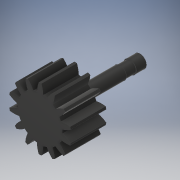
# Autodesk Inventor part: AC06
Saved by Autodesk Inventor 2017 (Build 210142000, 142)
## iProperties
Created: 2019-09-22
Part Number: AC06
Material: ABS Plastic
Document SubType Name: Modeling
Designer: Zach
Density: 1.06 g/cm^3
Appearance: Smooth - Black
Author: Zach
Autodesk Inventor part; units mm, degrees
ref_plane "YZ Plane" through (0, 0, 0) normal (1, 0, 0) x (0, 1, 0)
ref_plane "XZ Plane" through (0, 0, 0) normal (0, 1, 0) x (-1, 0, 0)
ref_plane "XY Plane" through (0, 0, 0) normal (0, 0, 1) x (1, 0, 0)
sketch "Sketch1" plane through (0, 0, 0) normal (0, 0, 1) x (1, 0, 0)
  arc A0 (5.9892, 8.4411) -> (6.9584, 12.5904) centre (-5.202, 13.243) ccw
  arc A1 (6.9584, 12.5904) -> (5.505, 13.2903) centre (0, 0) ccw
  arc A2 (5.505, 13.2903) -> (2.8652, 9.9455) centre (13.5971, 4.1898) ccw
  arc A3 (2.8652, 9.9455) -> (1.7337, 10.2038) centre (0, 0) ccw
  arc A4 (1.7337, 10.2038) -> (0.8066, 14.3627) centre (-10.4327, 9.6744) ccw
  arc A5 (0.8066, 14.3627) -> (-0.8066, 14.3627) centre (0, 0) ccw
  arc A6 (-0.8066, 14.3627) -> (-1.7337, 10.2038) centre (10.4327, 9.6744) ccw
  arc A7 (-1.7337, 10.2038) -> (-2.8652, 9.9455) centre (0, 0) ccw
  arc A8 (-2.8652, 9.9455) -> (-5.505, 13.2903) centre (-13.5971, 4.1898) ccw
  arc A9 (-5.505, 13.2903) -> (-6.9584, 12.5904) centre (0, 0) ccw
  arc A10 (-6.9584, 12.5904) -> (-5.9892, 8.4411) centre (5.202, 13.243) ccw
  arc A11 (-5.9892, 8.4411) -> (-6.8967, 7.7174) centre (0, 0) ccw
  arc A12 (-6.8967, 7.7174) -> (-10.7263, 9.5856) centre (-14.0685, -2.1247) ccw
  arc A13 (-10.7263, 9.5856) -> (-11.7321, 8.3244) centre (0, 0) ccw
  arc A14 (-11.7321, 8.3244) -> (-9.0586, 5.0065) centre (-1.0591, 14.1885) ccw
  arc A15 (-9.0586, 5.0065) -> (-9.5622, 3.9608) centre (0, 0) ccw
  arc A16 (-9.5622, 3.9608) -> (-13.8231, 3.9824) centre (-11.7534, -8.0184) ccw
  arc A17 (-13.8231, 3.9824) -> (-14.1821, 2.4096) centre (0, 0) ccw
  arc A18 (-14.1821, 2.4096) -> (-10.3337, 0.5803) centre (-7.1104, 12.3239) ccw
  arc A19 (-10.3337, 0.5803) -> (-10.3337, -0.5803) centre (0, 0) ccw
  arc A20 (-10.3337, -0.5803) -> (-14.1821, -2.4096) centre (-7.1104, -12.3239) ccw
  arc A21 (-14.1821, -2.4096) -> (-13.8231, -3.9824) centre (0, 0) ccw
  arc A22 (-13.8231, -3.9824) -> (-9.5622, -3.9608) centre (-11.7534, 8.0184) ccw
  arc A23 (-9.5622, -3.9608) -> (-9.0586, -5.0065) centre (0, 0) ccw
  arc A24 (-9.0586, -5.0065) -> (-11.7321, -8.3244) centre (-1.0591, -14.1885) ccw
  arc A25 (-11.7321, -8.3244) -> (-10.7263, -9.5856) centre (0, 0) ccw
  arc A26 (-10.7263, -9.5856) -> (-6.8967, -7.7174) centre (-14.0685, 2.1247) ccw
  arc A27 (-6.8967, -7.7174) -> (-5.9892, -8.4411) centre (0, 0) ccw
  arc A28 (-5.9892, -8.4411) -> (-6.9584, -12.5904) centre (5.202, -13.243) ccw
  arc A29 (-6.9584, -12.5904) -> (-5.505, -13.2903) centre (0, 0) ccw
  arc A30 (-5.505, -13.2903) -> (-2.8652, -9.9455) centre (-13.5971, -4.1898) ccw
  arc A31 (-2.8652, -9.9455) -> (-1.7337, -10.2038) centre (0, 0) ccw
  arc A32 (-1.7337, -10.2038) -> (-0.8066, -14.3627) centre (10.4327, -9.6744) ccw
  arc A33 (-0.8066, -14.3627) -> (0.8066, -14.3627) centre (0, 0) ccw
  arc A34 (0.8066, -14.3627) -> (1.7337, -10.2038) centre (-10.4327, -9.6744) ccw
  arc A35 (1.7337, -10.2038) -> (2.8652, -9.9455) centre (0, 0) ccw
  arc A36 (2.8652, -9.9455) -> (5.505, -13.2903) centre (13.5971, -4.1898) ccw
  arc A37 (5.505, -13.2903) -> (6.9584, -12.5904) centre (0, 0) ccw
  arc A38 (6.9584, -12.5904) -> (5.9892, -8.4411) centre (-5.202, -13.243) ccw
  arc A39 (5.9892, -8.4411) -> (6.8967, -7.7174) centre (0, 0) ccw
  arc A40 (6.8967, -7.7174) -> (10.7263, -9.5856) centre (14.0685, 2.1247) ccw
  arc A41 (10.7263, -9.5856) -> (11.7321, -8.3244) centre (0, 0) ccw
  arc A42 (11.7321, -8.3244) -> (9.0586, -5.0065) centre (1.0591, -14.1885) ccw
  arc A43 (9.0586, -5.0065) -> (9.5622, -3.9608) centre (0, 0) ccw
  arc A44 (9.5622, -3.9608) -> (13.8231, -3.9824) centre (11.7534, 8.0184) ccw
  arc A45 (13.8231, -3.9824) -> (14.1821, -2.4096) centre (0, 0) ccw
  arc A46 (14.1821, -2.4096) -> (10.3337, -0.5803) centre (7.1104, -12.3239) ccw
  arc A47 (10.3337, -0.5803) -> (10.3337, 0.5803) centre (0, 0) ccw
  arc A48 (10.3337, 0.5803) -> (14.1821, 2.4096) centre (7.1104, 12.3239) ccw
  arc A49 (14.1821, 2.4096) -> (13.8231, 3.9824) centre (0, 0) ccw
  arc A50 (13.8231, 3.9824) -> (9.5622, 3.9608) centre (11.7534, -8.0184) ccw
  arc A51 (9.5622, 3.9608) -> (9.0586, 5.0065) centre (0, 0) ccw
  arc A52 (9.0586, 5.0065) -> (11.7321, 8.3244) centre (1.0591, 14.1885) ccw
  arc A53 (11.7321, 8.3244) -> (10.7263, 9.5856) centre (0, 0) ccw
  arc A54 (10.7263, 9.5856) -> (6.8967, 7.7174) centre (14.0685, -2.1247) ccw
  arc A55 (6.8967, 7.7174) -> (5.9892, 8.4411) centre (0, 0) ccw
  constraints: 112 point on circle, 56 centre point
extrude "Extrusion1" add sketch "Sketch1" along normal blind 16
sketch "Sketch2" plane through (0, 0, 0) normal (0, 0, -1) x (-1, 0, 0)
  circle A0 centre (0, 0) radius 2.925
  dimension "d2" = 5.85
  constraints: 1 centre point, 1 coincident
  measures "d2" diameter of A0
extrude "Extrusion2" add sketch "Sketch2" along normal blind 20
sketch "Sketch4" plane through (0, 0, -20) normal (0, 0, -1) x (-1, 0, 0)
  circle A0 centre (0, 0) radius 2.675
  dimension "d8" = 5.35
  constraints: 1 centre point, 1 coincident
  measures "d8" diameter of A0
extrude "Extrusion4" add sketch "Sketch4" along normal blind 4.5
sketch "Sketch7" plane through (0, 0, -24.5) normal (0, 0, -1) x (-1, 0, 0)
  circle A0 centre (0, 0) radius 2.925 projected
extrude "Extrusion6" add sketch "Sketch7" along normal blind 4.5
sketch "Sketch10" plane through (0, 0, 16) normal (0, 0, 1) x (1, 0, 0)
  arc A0 (10.7263, 9.5856) -> (6.8967, 7.7174) centre (14.0685, -2.1247) ccw projected
  arc A1 (6.8967, 7.7174) -> (5.9892, 8.4411) centre (0, 0) ccw projected
  arc A2 (5.9892, 8.4411) -> (6.9584, 12.5904) centre (-5.202, 13.243) ccw projected
  arc A3 (6.9584, 12.5904) -> (5.505, 13.2903) centre (0, 0) ccw projected
  arc A4 (5.505, 13.2903) -> (2.8652, 9.9455) centre (13.5971, 4.1898) ccw projected
  arc A5 (2.8652, 9.9455) -> (1.7337, 10.2038) centre (0, 0) ccw projected
  arc A6 (1.7337, 10.2038) -> (0.8066, 14.3627) centre (-10.4327, 9.6744) ccw projected
  arc A7 (0.8066, 14.3627) -> (-0.8066, 14.3627) centre (0, 0) ccw projected
  arc A8 (-0.8066, 14.3627) -> (-1.7337, 10.2038) centre (10.4327, 9.6744) ccw projected
  arc A9 (-1.7337, 10.2038) -> (-2.8652, 9.9455) centre (0, 0) ccw projected
  arc A10 (-2.8652, 9.9455) -> (-5.505, 13.2903) centre (-13.5971, 4.1898) ccw projected
  arc A11 (-5.505, 13.2903) -> (-6.9584, 12.5904) centre (0, 0) ccw projected
  arc A12 (-6.9584, 12.5904) -> (-5.9892, 8.4411) centre (5.202, 13.243) ccw projected
  arc A13 (-5.9892, 8.4411) -> (-6.8967, 7.7174) centre (0, 0) ccw projected
  arc A14 (-6.8967, 7.7174) -> (-10.7263, 9.5856) centre (-14.0685, -2.1247) ccw projected
  arc A15 (-10.7263, 9.5856) -> (-11.7321, 8.3244) centre (0, 0) ccw projected
  arc A16 (-11.7321, 8.3244) -> (-9.0586, 5.0065) centre (-1.0591, 14.1885) ccw projected
  arc A17 (-9.0586, 5.0065) -> (-9.5622, 3.9608) centre (0, 0) ccw projected
  arc A18 (-9.5622, 3.9608) -> (-13.8231, 3.9824) centre (-11.7534, -8.0184) ccw projected
  arc A19 (-13.8231, 3.9824) -> (-14.1821, 2.4096) centre (0, 0) ccw projected
  arc A20 (-14.1821, 2.4096) -> (-10.3337, 0.5803) centre (-7.1104, 12.3239) ccw projected
  arc A21 (-10.3337, 0.5803) -> (-10.3337, -0.5803) centre (0, 0) ccw projected
  arc A22 (-10.3337, -0.5803) -> (-14.1821, -2.4096) centre (-7.1104, -12.3239) ccw projected
  arc A23 (-14.1821, -2.4096) -> (-13.8231, -3.9824) centre (0, 0) ccw projected
  arc A24 (-13.8231, -3.9824) -> (-9.5622, -3.9608) centre (-11.7534, 8.0184) ccw projected
  arc A25 (-9.5622, -3.9608) -> (-9.0586, -5.0065) centre (0, 0) ccw projected
  arc A26 (-9.0586, -5.0065) -> (-11.7321, -8.3244) centre (-1.0591, -14.1885) ccw projected
  arc A27 (-11.7321, -8.3244) -> (-10.7263, -9.5856) centre (0, 0) ccw projected
  arc A28 (-10.7263, -9.5856) -> (-6.8967, -7.7174) centre (-14.0685, 2.1247) ccw projected
  arc A29 (-6.8967, -7.7174) -> (-5.9892, -8.4411) centre (0, 0) ccw projected
  arc A30 (-5.9892, -8.4411) -> (-6.9584, -12.5904) centre (5.202, -13.243) ccw projected
  arc A31 (-6.9584, -12.5904) -> (-5.505, -13.2903) centre (0, 0) ccw projected
  arc A32 (-5.505, -13.2903) -> (-2.8652, -9.9455) centre (-13.5971, -4.1898) ccw projected
  arc A33 (-2.8652, -9.9455) -> (-1.7337, -10.2038) centre (0, 0) ccw projected
  arc A34 (-1.7337, -10.2038) -> (-0.8066, -14.3627) centre (10.4327, -9.6744) ccw projected
  arc A35 (-0.8066, -14.3627) -> (0.8066, -14.3627) centre (0, 0) ccw projected
  arc A36 (0.8066, -14.3627) -> (1.7337, -10.2038) centre (-10.4327, -9.6744) ccw projected
  arc A37 (1.7337, -10.2038) -> (2.8652, -9.9455) centre (0, 0) ccw projected
  arc A38 (2.8652, -9.9455) -> (5.505, -13.2903) centre (13.5971, -4.1898) ccw projected
  arc A39 (5.505, -13.2903) -> (6.9584, -12.5904) centre (0, 0) ccw projected
  arc A40 (6.9584, -12.5904) -> (5.9892, -8.4411) centre (-5.202, -13.243) ccw projected
  arc A41 (5.9892, -8.4411) -> (6.8967, -7.7174) centre (0, 0) ccw projected
  arc A42 (6.8967, -7.7174) -> (10.7263, -9.5856) centre (14.0685, 2.1247) ccw projected
  arc A43 (10.7263, -9.5856) -> (11.7321, -8.3244) centre (0, 0) ccw projected
  arc A44 (11.7321, -8.3244) -> (9.0586, -5.0065) centre (1.0591, -14.1885) ccw projected
  arc A45 (9.0586, -5.0065) -> (9.5622, -3.9608) centre (0, 0) ccw projected
  arc A46 (9.5622, -3.9608) -> (13.8231, -3.9824) centre (11.7534, 8.0184) ccw projected
  arc A47 (13.8231, -3.9824) -> (14.1821, -2.4096) centre (0, 0) ccw projected
  arc A48 (14.1821, -2.4096) -> (10.3337, -0.5803) centre (7.1104, -12.3239) ccw projected
  arc A49 (10.3337, -0.5803) -> (10.3337, 0.5803) centre (0, 0) ccw projected
  arc A50 (10.3337, 0.5803) -> (14.1821, 2.4096) centre (7.1104, 12.3239) ccw projected
  arc A51 (14.1821, 2.4096) -> (13.8231, 3.9824) centre (0, 0) ccw projected
  arc A52 (13.8231, 3.9824) -> (9.5622, 3.9608) centre (11.7534, -8.0184) ccw projected
  arc A53 (9.5622, 3.9608) -> (9.0586, 5.0065) centre (0, 0) ccw projected
  arc A54 (9.0586, 5.0065) -> (11.7321, 8.3244) centre (1.0591, 14.1885) ccw projected
  arc A55 (11.7321, 8.3244) -> (10.7263, 9.5856) centre (0, 0) ccw projected
  arc A56 (0.5421, 13.9895) -> (-0.5421, 13.9895) centre (0, 0) ccw
  arc A57 (1.3582, 9.8717) -> (0.5421, 13.9895) centre (-10.4327, 9.6744) ccw
  arc A58 (3.0594, 9.4834) -> (1.3582, 9.8717) centre (0, 0) ccw
  arc A59 (5.5814, 12.8393) -> (3.0594, 9.4834) centre (13.5971, 4.1898) ccw
  arc A60 (6.5582, 12.3689) -> (5.5814, 12.8393) centre (0, 0) ccw
  arc A61 (5.5069, 8.3048) -> (6.5582, 12.3689) centre (-5.202, 13.243) ccw
  arc A62 (6.8711, 7.2168) -> (5.5069, 8.3048) centre (0, 0) ccw
  arc A63 (10.5995, 9.1461) -> (6.8711, 7.2168) centre (14.0685, -2.1247) ccw
  arc A64 (11.2754, 8.2985) -> (10.5995, 9.1461) centre (0, 0) ccw
  arc A65 (8.5648, 5.093) -> (11.2754, 8.2985) centre (1.0591, 14.1885) ccw
  arc A66 (9.3219, 3.5208) -> (8.5648, 5.093) centre (0, 0) ccw
  arc A67 (13.5181, 3.6414) -> (9.3219, 3.5208) centre (11.7534, -8.0184) ccw
  arc A68 (13.7594, 2.5845) -> (13.5181, 3.6414) centre (0, 0) ccw
  arc A69 (9.9264, 0.8725) -> (13.7594, 2.5845) centre (7.1104, 12.3239) ccw
  arc A70 (9.9264, -0.8725) -> (9.9264, 0.8725) centre (0, 0) ccw
  arc A71 (13.7594, -2.5845) -> (9.9264, -0.8725) centre (7.1104, -12.3239) ccw
  arc A72 (13.5181, -3.6414) -> (13.7594, -2.5845) centre (0, 0) ccw
  arc A73 (9.3219, -3.5208) -> (13.5181, -3.6414) centre (11.7534, 8.0184) ccw
  arc A74 (8.5648, -5.093) -> (9.3219, -3.5208) centre (0, 0) ccw
  arc A75 (11.2754, -8.2985) -> (8.5648, -5.093) centre (1.0591, -14.1885) ccw
  arc A76 (10.5995, -9.1461) -> (11.2754, -8.2985) centre (0, 0) ccw
  arc A77 (6.8711, -7.2168) -> (10.5995, -9.1461) centre (14.0685, 2.1247) ccw
  arc A78 (5.5069, -8.3048) -> (6.8711, -7.2168) centre (0, 0) ccw
  arc A79 (6.5582, -12.3689) -> (5.5069, -8.3048) centre (-5.202, -13.243) ccw
  arc A80 (5.5814, -12.8393) -> (6.5582, -12.3689) centre (0, 0) ccw
  arc A81 (3.0594, -9.4834) -> (5.5814, -12.8393) centre (13.5971, -4.1898) ccw
  arc A82 (1.3582, -9.8717) -> (3.0594, -9.4834) centre (0, 0) ccw
  arc A83 (0.5421, -13.9895) -> (1.3582, -9.8717) centre (-10.4327, -9.6744) ccw
  arc A84 (-0.5421, -13.9895) -> (0.5421, -13.9895) centre (0, 0) ccw
  arc A85 (-1.3582, -9.8717) -> (-0.5421, -13.9895) centre (10.4327, -9.6744) ccw
  arc A86 (-3.0594, -9.4834) -> (-1.3582, -9.8717) centre (0, 0) ccw
  arc A87 (-5.5814, -12.8393) -> (-3.0594, -9.4834) centre (-13.5971, -4.1898) ccw
  arc A88 (-6.5582, -12.3689) -> (-5.5814, -12.8393) centre (0, 0) ccw
  arc A89 (-5.5069, -8.3048) -> (-6.5582, -12.3689) centre (5.202, -13.243) ccw
  arc A90 (-6.8711, -7.2168) -> (-5.5069, -8.3048) centre (0, 0) ccw
  arc A91 (-10.5995, -9.1461) -> (-6.8711, -7.2168) centre (-14.0685, 2.1247) ccw
  arc A92 (-11.2754, -8.2985) -> (-10.5995, -9.1461) centre (0, 0) ccw
  arc A93 (-8.5648, -5.093) -> (-11.2754, -8.2985) centre (-1.0591, -14.1885) ccw
  arc A94 (-9.3219, -3.5208) -> (-8.5648, -5.093) centre (0, 0) ccw
  arc A95 (-13.5181, -3.6414) -> (-9.3219, -3.5208) centre (-11.7534, 8.0184) ccw
  arc A96 (-13.7594, -2.5845) -> (-13.5181, -3.6414) centre (0, 0) ccw
  arc A97 (-9.9264, -0.8725) -> (-13.7594, -2.5845) centre (-7.1104, -12.3239) ccw
  arc A98 (-9.9264, 0.8725) -> (-9.9264, -0.8725) centre (0, 0) ccw
  arc A99 (-13.7594, 2.5845) -> (-9.9264, 0.8725) centre (-7.1104, 12.3239) ccw
  arc A100 (-13.5181, 3.6414) -> (-13.7594, 2.5845) centre (0, 0) ccw
  arc A101 (-9.3219, 3.5208) -> (-13.5181, 3.6414) centre (-11.7534, -8.0184) ccw
  arc A102 (-8.5648, 5.093) -> (-9.3219, 3.5208) centre (0, 0) ccw
  arc A103 (-11.2754, 8.2985) -> (-8.5648, 5.093) centre (-1.0591, 14.1885) ccw
  arc A104 (-10.5995, 9.1461) -> (-11.2754, 8.2985) centre (0, 0) ccw
  arc A105 (-6.8711, 7.2168) -> (-10.5995, 9.1461) centre (-14.0685, -2.1247) ccw
  arc A106 (-5.5069, 8.3048) -> (-6.8711, 7.2168) centre (0, 0) ccw
  arc A107 (-6.5582, 12.3689) -> (-5.5069, 8.3048) centre (5.202, 13.243) ccw
  arc A108 (-5.5814, 12.8393) -> (-6.5582, 12.3689) centre (0, 0) ccw
  arc A109 (-3.0594, 9.4834) -> (-5.5814, 12.8393) centre (-13.5971, 4.1898) ccw
  arc A110 (-1.3582, 9.8717) -> (-3.0594, 9.4834) centre (0, 0) ccw
  arc A111 (-0.5421, 13.9895) -> (-1.3582, 9.8717) centre (10.4327, 9.6744) ccw
  dimension "d20" = 14
  constraints: 112 point on circle, 56 centre point, 55 other
  measures "d20" radius of A56
extrude "Extrusion8" cut sketch "Sketch10" against normal through all
body "Solid1"
